Casing v4 (Autodesk Fusion 360 design; units mm, degrees)
Autodesk Fusion 360 part; units mm, degrees
note: some values were not read from the file. Set by a fixed rule: which face or edge a step refers to.
sketch "Sketch1" plane through (0, 0, 0) normal (0, 1, 0) x (1, 0, 0)
  circle A0 centre (0, 0) radius 37.5
  circle A1 centre (0, 0) radius 33.6
  dimension "d1" = 75
  dimension "d2" = 67.2
  constraint coincident A0.centre A1.centre
  measures "d1" diameter of A0
  measures "d2" diameter of A1
extrude "Extrude1" add sketch "Sketch1" along normal mid plane 120
thread "Thread1" "ISO Metric profile 68.0 M68x4 6H" major diameter 68.4462 minor diameter 63.9699 pitch 4 angle 60 modelled right hand crest width 1.0823 on face at (33.433, 40, 3.3455) from (0, 40, 0) to (0, 60, 0) crest through (31.985, -59, 0)
sketch "Sketch2" plane through (0, -60, 0) normal (0, -1, 0) x (1, 0, 0)
  circle A0 centre (0, 0) radius 31.985
  circle A1 centre (0, 0) radius 37.5
extrude "Extrude2" add sketch "Sketch2" along normal blind 5 contours A0 | A1
sketch "Sketch3" plane through (0, 0, 0) normal (0, 0, 1) x (1, 0, 0)
  line L0 (-37.5, -65) -> (37.5, -65)
  ellipse E0 centre (0, -65) end of major axis (-37.5, -65) minor radius 25 (-37.5, -65) -> (0, -90) ccw
  line L1 (0, -65) -> (0, -90)
  dimension "d9" = 50
  constraint midpoint L0 E0.centre
  constraint coincident E0.centre L1.start
  constraint perpendicular L0 L1
revolve "Revolve1" add sketch "Sketch3" angle 360 about axis through (0, -65, 0) along (0, -1, 0)
sketch "Sketch4" plane through (0, 0, 0) normal (0, 1, 0) x (1, 0, 0)
  line L0 (-40, 15) -> (-35, 15)
  line L1 (-35, 15) -> (-35, -15)
  line L2 (-35, -15) -> (-40, -15)
  line L3 (-40, -15) -> (-40, 15)
  line L4 (-35, -15) -> (-40, 15) construction
  line L5 (-35, 15) -> (-40, -15) construction
  line L6 (-37.5, 0) -> (0, 0) construction
  circle A0 centre (0, 0) radius 37.5 construction
  point P0 (-37.5, 0)
  dimension "d11" = 5
  dimension "d12" = 30
  constraint horizontal L0
  constraint vertical L1
  constraint horizontal L2
  constraint vertical L3
  constraint midpoint L4 P0
  constraint coincident P0 L6.start
  constraint coincident L6.end A0.centre
  constraint horizontal L6
  constraint coincident P0 A0
  measures "d11" distance of L0.start L0.end
  measures "d12" distance of L0.start L2.end
extrude "Extrude3" cut sketch "Sketch4" along normal through all and the other way through all
pattern_circular "C-Pattern1" count 2 over 360 about axis through (0, -65, 0) along (0, 1, 0) of "Extrude3"
fillet "Fillet2" radius 0.5 2 edges at (-24.03, 50, -21.1084) (24.03, 50, -21.1084)
